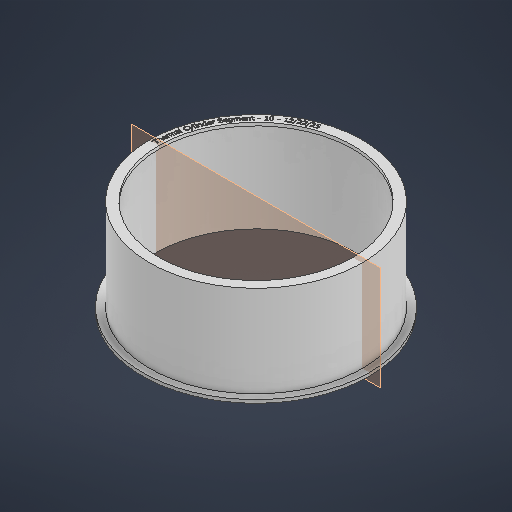
# Autodesk Inventor part: 10
Saved by Autodesk Inventor 2026.2 (Build 302298000, 298)
## iProperties
Created: 2024-04-11
Part Number: 10
Material: Generic
Document SubType Name: Modeling
Designer: Thienan Hoang
Density: 1 g/cm^3
Appearance: Default
Author: Thienan Hoang
Autodesk Inventor part; units mm, degrees
ref_plane "YZ Plane" through (0, 0, 0) normal (1, 0, 0) x (0, 1, 0)
ref_plane "XZ Plane" through (0, 0, 0) normal (0, 1, 0) x (-1, 0, 0)
sketch "Sketch1" plane through (0, 0, 0) normal (0, 1, 0) x (-1, 0, 0)
  circle A0 centre (0, 0) radius 72
  circle A1 centre (0, 0) radius 67.5
  circle A2 centre (0, 0) radius 63.5
  dimension "Absolute_Diameter" = 144
  dimension "Diameter_No_Outer_Lip" = 135
  dimension "Inner_Cylinder_Diameter" = 127
  constraints: 3 centre point, 3 coincident
  measures "Absolute_Diameter" diameter of A0
  measures "Diameter_No_Outer_Lip" diameter of A1
  measures "Inner_Cylinder_Diameter" diameter of A2
extrude "Extrusion1" add sketch "Sketch1" along normal blind 2 contours A0
extrude "Extrusion2" add sketch "Sketch1" along normal blind 60 contours A1
sketch "Sketch2" plane through (0, 60, 0) normal (0, 1, 0) x (1, 0, 0)
  circle A0 centre (0, 0) radius 61.5
  circle A1 centre (0, 0) radius 66.5
  dimension "Lip_Diameter_Out" = 123
  dimension "Top_Outer_Lip_Diameter" = 133
  constraints: 2 centre point, 2 coincident
  measures "Lip_Diameter_Out" diameter of A0
  measures "Top_Outer_Lip_Diameter" diameter of A1
extrude "Extrusion7" add sketch "Sketch2" against normal blind 2
ref_plane "Work Plane2" through (0, 10, 0) normal (0, 1, 0) x (1, 0, 0)
sketch "Sketch3" plane through (0, 10, 0) normal (0, 1, 0) x (1, 0, 0)
  circle A0 centre (0, 0) radius 127.5
  circle A1 centre (-127.5, 0) radius 2.5
  circle A2 centre (-103.1497, -74.9426) radius 2.5
  circle A3 centre (-39.3997, -121.2597) radius 2.5
  circle A4 centre (39.3997, -121.2597) radius 2.5
  circle A5 centre (103.1497, -74.9426) radius 2.5
  circle A6 centre (127.5, 0) radius 2.5
  circle A7 centre (103.1497, 74.9426) radius 2.5
  circle A8 centre (39.3997, 121.2597) radius 2.5
  circle A9 centre (-39.3997, 121.2597) radius 2.5
  circle A10 centre (-103.1497, 74.9426) radius 2.5
  dimension "d27" = 255
  dimension "d28" = 5
  dimension "d31" = 360
  constraints: 10 centre point, 1 coincident, 1 horizontal alignment, 23 other
  measures "d28" diameter of A1
extrude "Extrusion8" [suppressed]
sketch "Sketch24" plane through (0, 60, 0) normal (0, 1, 0) x (1, 0, 0)
  circle A0 centre (0, 0) radius 51
  circle A1 centre (0, -51) radius 2.75
  circle A2 centre (44.1673, -25.5) radius 2.75
  circle A3 centre (44.1673, 25.5) radius 2.75
  circle A4 centre (0, 51) radius 2.75
  circle A5 centre (-44.1673, 25.5) radius 2.75
  circle A6 centre (-44.1673, -25.5) radius 2.75
  dimension "d230" = 102
  dimension "d231" = 5.5
  dimension "d234" = 360
  constraints: 6 centre point, 1 coincident, 1 vertical alignment, 15 other
  measures "d231" diameter of A1
extrude "Extrusion30" [suppressed]
sketch "Sketch48" plane through (0, 60, 0) normal (0, 1, 0) x (1, 0, 0)
  circle A0 centre (0, 0) radius 58.25
  line L0 (-63.2421, 1.0199) -> (-65.929, 1.072)
  line L1 (-65.929, 1.072) -> (-65.9488, 0.0496)
  line L2 (-65.9488, 0.0496) -> (-66.3093, 0.0566)
  line L3 (-66.3093, 0.0566) -> (-66.2619, 2.5064)
  line L4 (-66.2619, 2.5064) -> (-65.9013, 2.4994)
  line L5 (-65.9013, 2.4994) -> (-65.9211, 1.477)
  line L6 (-65.9211, 1.477) -> (-63.2343, 1.4249)
  line L7 (-63.2343, 1.4249) -> (-63.2421, 1.0199)
  line L8 (-63.0947, 4.5212) -> (-63.1167, 4.1365)
  line L9 (-63.1167, 4.1365) -> (-64.4188, 4.211)
  spline S0 degree 2 poles (-64.4188, 4.211) (-64.5766, 4.2201) (-64.8496, 4.206) (-64.9335, 4.1663) knots 0 0 0 1 2 2 2
  spline S1 degree 2 poles (-64.9335, 4.1663) (-65.0225, 4.1244) (-65.1159, 3.9615) (-65.1241, 3.8185) knots 0 0 0 1 2 2 2
  spline S2 degree 2 poles (-65.1241, 3.8185) (-65.1323, 3.6754) (-64.9968, 3.3634) (-64.8818, 3.2108) knots 0 0 0 1 2 2 2
  line L10 (-64.8818, 3.2108) -> (-63.1754, 3.1131)
  line L11 (-63.1754, 3.1131) -> (-63.1974, 2.7284)
  line L12 (-63.1974, 2.7284) -> (-66.376, 2.9104)
  line L13 (-66.376, 2.9104) -> (-66.354, 3.2951)
  line L14 (-66.354, 3.2951) -> (-65.2048, 3.2293)
  spline S3 degree 2 poles (-65.2048, 3.2293) (-65.3503, 3.4108) (-65.494, 3.7531) (-65.4833, 3.9405) knots 0 0 0 1 2 2 2
  spline S4 degree 2 poles (-65.4833, 3.9405) (-65.4641, 4.2759) (-64.9984, 4.6302) (-64.5768, 4.606) knots 0 0 0 1 2 2 2
  line L15 (-64.5768, 4.606) -> (-63.0947, 4.5212)
  spline S5 degree 2 poles (-62.9087, 6.0442) (-62.9596, 5.4982) (-63.628, 4.9553) (-64.1937, 5.0082) knots 0 0 0 1 2 2 2
  spline S6 degree 2 poles (-64.1937, 5.0082) (-64.7495, 5.0601) (-65.3542, 5.7045) (-65.3103, 6.1742) knots 0 0 0 1 2 2 2
  spline S7 degree 2 poles (-65.3103, 6.1742) (-65.2906, 6.3857) (-65.137, 6.7013) (-64.9955, 6.8096) knots 0 0 0 1 2 2 2
  spline S8 degree 2 poles (-64.9955, 6.8096) (-64.8536, 6.9204) (-64.4652, 7.0156) (-64.1922, 6.9902) knots 0 0 0 1 2 2 2
  line L16 (-64.1922, 6.9902) -> (-63.9832, 6.9706)
  line L17 (-63.9832, 6.9706) -> (-64.1304, 5.3942)
  spline S9 degree 2 poles (-64.1304, 5.3942) (-63.7344, 5.3572) (-63.2767, 5.7164) (-63.2436, 6.0705) knots 0 0 0 1 2 2 2
  spline S10 degree 2 poles (-63.2436, 6.0705) (-63.2319, 6.1959) (-63.2657, 6.4447) (-63.3008, 6.5472) knots 0 0 0 1 2 2 2
  spline S11 degree 2 poles (-63.3008, 6.5472) (-63.3403, 6.6551) (-63.4131, 6.8058) (-63.4481, 6.8562) knots 0 0 0 1 2 2 2
  line L18 (-63.4481, 6.8562) -> (-63.446, 6.8783)
  line L19 (-63.446, 6.8783) -> (-63.0279, 6.8393)
  spline S12 degree 2 poles (-63.0279, 6.8393) (-63.0071, 6.7703) (-62.9472, 6.5613) (-62.9324, 6.4806) knots 0 0 0 1 2 2 2
  spline S13 degree 2 poles (-62.9324, 6.4806) (-62.9108, 6.3669) (-62.8958, 6.1819) (-62.9087, 6.0442) knots 0 0 0 1 2 2 2
  spline S14 degree 2 poles (-64.3107, 6.6241) (-64.4661, 6.6337) (-64.6983, 6.5909) (-64.7803, 6.5365) knots 0 0 0 1 2 2 2
  spline S15 degree 2 poles (-64.7803, 6.5365) (-64.8726, 6.4782) (-64.9831, 6.2776) (-64.9976, 6.1227) knots 0 0 0 1 2 2 2
  spline S16 degree 2 poles (-64.9976, 6.1227) (-65.0118, 5.9702) (-64.9408, 5.7477) (-64.8605, 5.6509) knots 0 0 0 1 2 2 2
  spline S17 degree 2 poles (-64.8605, 5.6509) (-64.7776, 5.5564) (-64.567, 5.4474) (-64.423, 5.4215) knots 0 0 0 1 2 2 2
  line L20 (-64.423, 5.4215) -> (-64.3107, 6.6241)
  line L21 (-64.5468, 8.6879) -> (-64.5493, 8.6683)
  spline S18 degree 2 poles (-64.5493, 8.6683) (-64.5669, 8.6256) (-64.5836, 8.5306) (-64.5918, 8.4644) knots 0 0 0 1 2 2 2
  spline S19 degree 2 poles (-64.5918, 8.4644) (-64.6108, 8.31) (-64.5134, 7.9894) (-64.3979, 7.8358) knots 0 0 0 1 2 2 2
  line L22 (-64.3979, 7.8358) -> (-62.7873, 7.6375)
  line L23 (-62.7873, 7.6375) -> (-62.8343, 7.2551)
  line L24 (-62.8343, 7.2551) -> (-65.1044, 7.5346)
  line L25 (-65.1044, 7.5346) -> (-65.0573, 7.917)
  line L26 (-65.0573, 7.917) -> (-64.719, 7.8754)
  spline S20 degree 2 poles (-64.719, 7.8754) (-64.8797, 8.1067) (-64.9934, 8.4367) (-64.9753, 8.5838) knots 0 0 0 1 2 2 2
  spline S21 degree 2 poles (-64.9753, 8.5838) (-64.968, 8.6427) (-64.9559, 8.7009) (-64.944, 8.7368) knots 0 0 0 1 2 2 2
  line L27 (-64.944, 8.7368) -> (-64.5468, 8.6879)
  line L28 (-62.2395, 11.316) -> (-63.546, 11.5299)
  spline S22 degree 2 poles (-63.546, 11.5299) (-63.702, 11.5554) (-63.9717, 11.5745) (-64.0512, 11.5475) knots 0 0 0 1 2 2 2
  spline S23 degree 2 poles (-64.0512, 11.5475) (-64.138, 11.5217) (-64.2404, 11.3857) (-64.2615, 11.2565) knots 0 0 0 1 2 2 2
  spline S24 degree 2 poles (-64.2615, 11.2565) (-64.2807, 11.1395) (-64.1807, 10.8479) (-64.0674, 10.6841) knots 0 0 0 1 2 2 2
  spline S25 degree 2 poles (-64.0674, 10.6841) (-64.0328, 10.681) (-63.937, 10.6703) (-63.8736, 10.6599) knots 0 0 0 1 2 2 2
  line L29 (-63.8736, 10.6599) -> (-62.3867, 10.4165)
  line L30 (-62.3867, 10.4165) -> (-62.4489, 10.0363)
  line L31 (-62.4489, 10.0363) -> (-63.7555, 10.2501)
  spline S26 degree 2 poles (-63.7555, 10.2501) (-63.9115, 10.2757) (-64.1812, 10.2948) (-64.2607, 10.2678) knots 0 0 0 1 2 2 2
  spline S27 degree 2 poles (-64.2607, 10.2678) (-64.3475, 10.2419) (-64.4498, 10.106) (-64.471, 9.9768) knots 0 0 0 1 2 2 2
  spline S28 degree 2 poles (-64.471, 9.9768) (-64.4909, 9.8549) (-64.3817, 9.5592) (-64.283, 9.4129) knots 0 0 0 1 2 2 2
  line L32 (-64.283, 9.4129) -> (-62.5962, 9.1368)
  line L33 (-62.5962, 9.1368) -> (-62.6584, 8.7565)
  line L34 (-62.6584, 8.7565) -> (-64.9156, 9.126)
  line L35 (-64.9156, 9.126) -> (-64.8534, 9.5063)
  line L36 (-64.8534, 9.5063) -> (-64.6047, 9.4656)
  spline S29 degree 2 poles (-64.6047, 9.4656) (-64.7291, 9.6386) (-64.8445, 9.9579) (-64.8158, 10.1334) knots 0 0 0 1 2 2 2
  spline S30 degree 2 poles (-64.8158, 10.1334) (-64.7831, 10.3333) (-64.5496, 10.6129) (-64.3292, 10.6594) knots 0 0 0 1 2 2 2
  spline S31 degree 2 poles (-64.3292, 10.6594) (-64.4935, 10.864) (-64.6374, 11.223) (-64.6063, 11.4131) knots 0 0 0 1 2 2 2
  spline S32 degree 2 poles (-64.6063, 11.4131) (-64.5824, 11.5594) (-64.4531, 11.7835) (-64.3363, 11.8545) knots 0 0 0 1 2 2 2
  spline S33 degree 2 poles (-64.3363, 11.8545) (-64.2192, 11.9279) (-63.8957, 11.9776) (-63.6641, 11.9396) knots 0 0 0 1 2 2 2
  line L37 (-63.6641, 11.9396) -> (-62.1772, 11.6962)
  line L38 (-62.1772, 11.6962) -> (-62.2395, 11.316)
  spline S34 degree 2 poles (-62.0371, 13.522) (-62.0129, 13.4689) (-61.9246, 13.2888) (-61.9037, 13.2087) knots 0 0 0 1 2 2 2
  spline S35 degree 2 poles (-61.9037, 13.2087) (-61.8713, 13.0984) (-61.8549, 12.9006) (-61.8905, 12.7314) knots 0 0 0 1 2 2 2
  spline S36 degree 2 poles (-61.8905, 12.7314) (-61.9195, 12.5936) (-62.0759, 12.3665) (-62.19, 12.2921) knots 0 0 0 1 2 2 2
  spline S37 degree 2 poles (-62.19, 12.2921) (-62.3007, 12.222) (-62.5943, 12.1702) (-62.7441, 12.2018) knots 0 0 0 1 2 2 2
  spline S38 degree 2 poles (-62.7441, 12.2018) (-62.9762, 12.2506) (-63.2637, 12.5156) (-63.3132, 12.7481) knots 0 0 0 1 2 2 2
  spline S39 degree 2 poles (-63.3132, 12.7481) (-63.3605, 12.955) (-63.3179, 13.4811) (-63.2722, 13.782) knots 0 0 0 1 2 2 2
  line L39 (-63.2722, 13.782) -> (-63.3447, 13.7972)
  spline S40 degree 2 poles (-63.3447, 13.7972) (-63.4753, 13.8247) (-63.654, 13.7791) (-63.7152, 13.7162) knots 0 0 0 1 2 2 2
  spline S41 degree 2 poles (-63.7152, 13.7162) (-63.7764, 13.6534) (-63.8491, 13.4516) (-63.8725, 13.3404) knots 0 0 0 1 2 2 2
  spline S42 degree 2 poles (-63.8725, 13.3404) (-63.9, 13.2099) (-63.8969, 12.8407) (-63.8591, 12.6485) knots 0 0 0 1 2 2 2
  line L40 (-63.8591, 12.6485) -> (-63.8637, 12.6268)
  line L41 (-63.8637, 12.6268) -> (-64.248, 12.7077)
  spline S43 degree 2 poles (-64.248, 12.7077) (-64.2552, 12.8177) (-64.2458, 13.2221) (-64.2056, 13.413) knots 0 0 0 1 2 2 2
  spline S44 degree 2 poles (-64.2056, 13.413) (-64.1567, 13.6451) (-64.0176, 13.9465) (-63.8968, 14.0523) knots 0 0 0 1 2 2 2
  spline S45 degree 2 poles (-63.8968, 14.0523) (-63.779, 14.1562) (-63.4611, 14.2155) (-63.2509, 14.1713) knots 0 0 0 1 2 2 2
  line L42 (-63.2509, 14.1713) -> (-61.7209, 13.8492)
  line L43 (-61.7209, 13.8492) -> (-61.8002, 13.4721)
  line L44 (-61.8002, 13.4721) -> (-62.0371, 13.522)
  line L45 (-62.3513, 13.5881) -> (-62.9725, 13.7189)
  spline S46 degree 2 poles (-62.9725, 13.7189) (-62.9889, 13.581) (-63.0338, 13.1639) (-63.0221, 13.0276) knots 0 0 0 1 2 2 2
  spline S47 degree 2 poles (-63.0221, 13.0276) (-63.0077, 12.8681) (-62.858, 12.6321) (-62.6888, 12.5965) knots 0 0 0 1 2 2 2
  spline S48 degree 2 poles (-62.6888, 12.5965) (-62.4954, 12.5558) (-62.2539, 12.7321) (-62.2101, 12.94) knots 0 0 0 1 2 2 2
  spline S49 degree 2 poles (-62.2101, 12.94) (-62.173, 13.1164) (-62.2642, 13.4385) (-62.3513, 13.5881) knots 0 0 0 1 2 2 2
  line L46 (-61.5046, 14.7574) -> (-61.5934, 14.3825)
  line L47 (-61.5934, 14.3825) -> (-64.6916, 15.1159)
  line L48 (-64.6916, 15.1159) -> (-64.6028, 15.4909)
  line L49 (-64.6028, 15.4909) -> (-61.5046, 14.7574)
  spline S50 degree 2 poles (-60.6572, 17.7329) (-60.7393, 17.4481) (-61.0704, 17.0217) (-61.3132, 16.9015) knots 0 0 0 1 2 2 2
  spline S51 degree 2 poles (-61.3132, 16.9015) (-61.5537, 16.7806) (-62.1788, 16.7525) (-62.549, 16.8592) knots 0 0 0 1 2 2 2
  spline S52 degree 2 poles (-62.549, 16.8592) (-62.9169, 16.9652) (-63.4087, 17.3101) (-63.5592, 17.5462) knots 0 0 0 1 2 2 2
  spline S53 degree 2 poles (-63.5592, 17.5462) (-63.7055, 17.7786) (-63.7739, 18.3176) (-63.6883, 18.6142) knots 0 0 0 1 2 2 2
  spline S54 degree 2 poles (-63.6883, 18.6142) (-63.6459, 18.7614) (-63.5287, 19.0078) (-63.464, 19.1074) knots 0 0 0 1 2 2 2
  spline S55 degree 2 poles (-63.464, 19.1074) (-63.4057, 19.1934) (-63.2611, 19.3651) (-63.1809, 19.4474) knots 0 0 0 1 2 2 2
  line L50 (-63.1809, 19.4474) -> (-62.711, 19.3119)
  line L51 (-62.711, 19.3119) -> (-62.7198, 19.2811)
  spline S56 degree 2 poles (-62.7198, 19.2811) (-62.7824, 19.2425) (-62.9618, 19.1194) (-63.0594, 19.0216) knots 0 0 0 1 2 2 2
  spline S57 degree 2 poles (-63.0594, 19.0216) (-63.1532, 18.9278) (-63.3075, 18.687) (-63.3568, 18.5161) knots 0 0 0 1 2 2 2
  spline S58 degree 2 poles (-63.3568, 18.5161) (-63.4108, 18.3286) (-63.353, 17.9495) (-63.2421, 17.7813) knots 0 0 0 1 2 2 2
  spline S59 degree 2 poles (-63.2421, 17.7813) (-63.1281, 17.6148) (-62.7145, 17.3464) (-62.432, 17.265) knots 0 0 0 1 2 2 2
  spline S60 degree 2 poles (-62.432, 17.265) (-62.1306, 17.1782) (-61.6546, 17.1978) (-61.4688, 17.2805) knots 0 0 0 1 2 2 2
  spline S61 degree 2 poles (-61.4688, 17.2805) (-61.2884, 17.3622) (-61.0462, 17.6496) (-60.9928, 17.8348) knots 0 0 0 1 2 2 2
  spline S62 degree 2 poles (-60.9928, 17.8348) (-60.9443, 18.0033) (-60.9446, 18.3144) (-60.9741, 18.4437) knots 0 0 0 1 2 2 2
  spline S63 degree 2 poles (-60.9741, 18.4437) (-61.0051, 18.5683) (-61.0874, 18.7643) (-61.1195, 18.8224) knots 0 0 0 1 2 2 2
  line L52 (-61.1195, 18.8224) -> (-61.1113, 18.8509)
  line L53 (-61.1113, 18.8509) -> (-60.6461, 18.7168)
  spline S64 degree 2 poles (-60.6461, 18.7168) (-60.629, 18.6065) (-60.5952, 18.4117) (-60.5921, 18.2797) knots 0 0 0 1 2 2 2
  spline S65 degree 2 poles (-60.5921, 18.2797) (-60.5864, 18.1392) (-60.6066, 17.9085) (-60.6572, 17.7329) knots 0 0 0 1 2 2 2
  line L54 (-61.9503, 21.409) -> (-59.3602, 19.2647)
  line L55 (-59.3602, 19.2647) -> (-59.4888, 18.8728)
  line L56 (-59.4888, 18.8728) -> (-60.2669, 19.5596)
  line L57 (-60.2669, 19.5596) -> (-62.5933, 19.4493)
  line L58 (-62.5933, 19.4493) -> (-62.4639, 19.8436)
  line L59 (-62.4639, 19.8436) -> (-60.6591, 19.9092)
  line L60 (-60.6591, 19.9092) -> (-62.0751, 21.0288)
  line L61 (-62.0751, 21.0288) -> (-61.9503, 21.409)
  line L62 (-59.5421, 21.3387) -> (-59.671, 20.9756)
  line L63 (-59.671, 20.9756) -> (-62.6714, 22.0406)
  line L64 (-62.6714, 22.0406) -> (-62.5425, 22.4037)
  line L65 (-62.5425, 22.4037) -> (-59.5421, 21.3387)
  line L66 (-59.2119, 22.2384) -> (-59.3463, 21.8773)
  line L67 (-59.3463, 21.8773) -> (-61.49, 22.6749)
  line L68 (-61.49, 22.6749) -> (-61.3556, 23.036)
  line L69 (-61.3556, 23.036) -> (-59.2119, 22.2384)
  line L70 (-61.7026, 23.1942) -> (-61.8551, 22.7844)
  line L71 (-61.8551, 22.7844) -> (-62.2301, 22.924)
  line L72 (-62.2301, 22.924) -> (-62.0776, 23.3337)
  line L73 (-62.0776, 23.3337) -> (-61.7026, 23.1942)
  line L74 (-58.3464, 24.4352) -> (-58.4902, 24.0777)
  line L75 (-58.4902, 24.0777) -> (-59.7002, 24.5642)
  spline S66 degree 2 poles (-59.7002, 24.5642) (-59.8469, 24.6231) (-60.11, 24.697) (-60.2022, 24.6861) knots 0 0 0 1 2 2 2
  spline S67 degree 2 poles (-60.2022, 24.6861) (-60.3, 24.6748) (-60.4405, 24.5503) (-60.494, 24.4174) knots 0 0 0 1 2 2 2
  spline S68 degree 2 poles (-60.494, 24.4174) (-60.5474, 24.2845) (-60.5186, 23.9455) (-60.4584, 23.7642) knots 0 0 0 1 2 2 2
  line L76 (-60.4584, 23.7642) -> (-58.8725, 23.1266)
  line L77 (-58.8725, 23.1266) -> (-59.0163, 22.7691)
  line L78 (-59.0163, 22.7691) -> (-61.1384, 23.6223)
  line L79 (-61.1384, 23.6223) -> (-60.9947, 23.9798)
  line L80 (-60.9947, 23.9798) -> (-60.7586, 23.8849)
  spline S69 degree 2 poles (-60.7586, 23.8849) (-60.8385, 24.1034) (-60.8654, 24.4736) (-60.7954, 24.6477) knots 0 0 0 1 2 2 2
  spline S70 degree 2 poles (-60.7954, 24.6477) (-60.6701, 24.9594) (-60.1156, 25.1465) (-59.7238, 24.9889) knots 0 0 0 1 2 2 2
  line L81 (-59.7238, 24.9889) -> (-58.3464, 24.4352)
  line L82 (-57.4194, 26.5395) -> (-57.5762, 26.1875)
  line L83 (-57.5762, 26.1875) -> (-57.7883, 26.282)
  spline S71 degree 2 poles (-57.7883, 26.282) (-57.7568, 26.1706) (-57.7198, 26.0108) (-57.7177, 25.9125) knots 0 0 0 1 2 2 2
  spline S72 degree 2 poles (-57.7177, 25.9125) (-57.7147, 25.822) (-57.7477, 25.6447) (-57.795, 25.5386) knots 0 0 0 1 2 2 2
  spline S73 degree 2 poles (-57.795, 25.5386) (-57.8713, 25.3671) (-58.1421, 25.1417) (-58.325, 25.1014) knots 0 0 0 1 2 2 2
  spline S74 degree 2 poles (-58.325, 25.1014) (-58.5079, 25.0612) (-58.9642, 25.1293) (-59.2282, 25.2469) knots 0 0 0 1 2 2 2
  spline S75 degree 2 poles (-59.2282, 25.2469) (-59.5035, 25.3695) (-59.8418, 25.6905) (-59.9377, 25.882) knots 0 0 0 1 2 2 2
  spline S76 degree 2 poles (-59.9377, 25.882) (-60.0218, 26.0574) (-60.0338, 26.4494) (-59.9544, 26.6276) knots 0 0 0 1 2 2 2
  spline S77 degree 2 poles (-59.9544, 26.6276) (-59.885, 26.7833) (-59.7116, 26.9845) (-59.5821, 27.081) knots 0 0 0 1 2 2 2
  line L84 (-59.5821, 27.081) -> (-60.4846, 27.483)
  line L85 (-60.4846, 27.483) -> (-60.3278, 27.835)
  line L86 (-60.3278, 27.835) -> (-57.4194, 26.5395)
  line L87 (-58.0839, 26.4136) -> (-59.291, 26.9513)
  spline S78 degree 2 poles (-59.291, 26.9513) (-59.4125, 26.8486) (-59.5523, 26.6621) (-59.6056, 26.5425) knots 0 0 0 1 2 2 2
  spline S79 degree 2 poles (-59.6056, 26.5425) (-59.7262, 26.2718) (-59.4568, 25.784) (-59.0732, 25.6132) knots 0 0 0 1 2 2 2
  spline S80 degree 2 poles (-59.0732, 25.6132) (-58.7031, 25.4483) (-58.2083, 25.5091) (-58.0927, 25.7686) knots 0 0 0 1 2 2 2
  spline S81 degree 2 poles (-58.0927, 25.7686) (-58.0314, 25.9062) (-58.0331, 26.2423) (-58.0839, 26.4136) knots 0 0 0 1 2 2 2
  spline S82 degree 2 poles (-56.6996, 27.914) (-56.9405, 27.4214) (-57.7577, 27.1501) (-58.2681, 27.3997) knots 0 0 0 1 2 2 2
  spline S83 degree 2 poles (-58.2681, 27.3997) (-58.7696, 27.6449) (-59.1071, 28.4616) (-58.8998, 28.8854) knots 0 0 0 1 2 2 2
  spline S84 degree 2 poles (-58.8998, 28.8854) (-58.8065, 29.0762) (-58.5513, 29.3171) (-58.3805, 29.3683) knots 0 0 0 1 2 2 2
  spline S85 degree 2 poles (-58.3805, 29.3683) (-58.2086, 29.4218) (-57.8116, 29.3734) (-57.5653, 29.2529) knots 0 0 0 1 2 2 2
  line L88 (-57.5653, 29.2529) -> (-57.3767, 29.1607)
  line L89 (-57.3767, 29.1607) -> (-58.0722, 27.7383)
  spline S86 degree 2 poles (-58.0722, 27.7383) (-57.715, 27.5637) (-57.1598, 27.7376) (-57.0035, 28.0571) knots 0 0 0 1 2 2 2
  spline S87 degree 2 poles (-57.0035, 28.0571) (-56.9482, 28.1703) (-56.8918, 28.4149) (-56.8883, 28.5232) knots 0 0 0 1 2 2 2
  spline S88 degree 2 poles (-56.8883, 28.5232) (-56.8871, 28.6381) (-56.9019, 28.8048) (-56.9168, 28.8643) knots 0 0 0 1 2 2 2
  line L90 (-56.9168, 28.8643) -> (-56.907, 28.8843)
  line L91 (-56.907, 28.8843) -> (-56.5298, 28.6998)
  spline S89 degree 2 poles (-56.5298, 28.6998) (-56.5347, 28.6279) (-56.5526, 28.4113) (-56.5674, 28.3305) knots 0 0 0 1 2 2 2
  spline S90 degree 2 poles (-56.5674, 28.3305) (-56.5874, 28.2165) (-56.6388, 28.0382) (-56.6996, 27.914) knots 0 0 0 1 2 2 2
  spline S91 degree 2 poles (-57.8057, 28.9525) (-57.9477, 29.0164) (-58.18, 29.0586) (-58.2759, 29.0367) knots 0 0 0 1 2 2 2
  spline S92 degree 2 poles (-58.2759, 29.0367) (-58.3829, 29.0148) (-58.5572, 28.8663) (-58.6256, 28.7265) knots 0 0 0 1 2 2 2
  spline S93 degree 2 poles (-58.6256, 28.7265) (-58.6928, 28.589) (-58.7051, 28.3558) (-58.6643, 28.2368) knots 0 0 0 1 2 2 2
  spline S94 degree 2 poles (-58.6643, 28.2368) (-58.6202, 28.119) (-58.4618, 27.9426) (-58.3363, 27.8675) knots 0 0 0 1 2 2 2
  line L92 (-58.3363, 27.8675) -> (-57.8057, 28.9525)
  line L93 (-57.2963, 30.9663) -> (-57.3055, 30.9488)
  spline S95 degree 2 poles (-57.3055, 30.9488) (-57.3371, 30.9152) (-57.3863, 30.8322) (-57.4174, 30.7732) knots 0 0 0 1 2 2 2
  spline S96 degree 2 poles (-57.4174, 30.7732) (-57.4898, 30.6355) (-57.5121, 30.3012) (-57.4585, 30.1167) knots 0 0 0 1 2 2 2
  line L94 (-57.4585, 30.1167) -> (-56.0222, 29.3613)
  line L95 (-56.0222, 29.3613) -> (-56.2016, 29.0202)
  line L96 (-56.2016, 29.0202) -> (-58.2259, 30.0849)
  line L97 (-58.2259, 30.0849) -> (-58.0465, 30.4259)
  line L98 (-58.0465, 30.4259) -> (-57.7448, 30.2673)
  spline S97 degree 2 poles (-57.7448, 30.2673) (-57.8133, 30.5405) (-57.8028, 30.8894) (-57.7338, 31.0206) knots 0 0 0 1 2 2 2
  spline S98 degree 2 poles (-57.7338, 31.0206) (-57.7062, 31.073) (-57.6742, 31.1232) (-57.6504, 31.1525) knots 0 0 0 1 2 2 2
  line L99 (-57.6504, 31.1525) -> (-57.2963, 30.9663)
  spline S99 degree 2 poles (-54.3606, 32.2276) (-54.5294, 31.943) (-54.8852, 31.6141) (-55.0748, 31.4882) knots 0 0 0 1 2 2 2
  line L100 (-55.0748, 31.4882) -> (-55.5124, 31.7477)
  line L101 (-55.5124, 31.7477) -> (-55.4973, 31.7732)
  spline S100 degree 2 poles (-55.4973, 31.7732) (-55.2338, 31.8495) (-54.7971, 32.1792) (-54.6774, 32.3811) knots 0 0 0 1 2 2 2
  spline S101 degree 2 poles (-54.6774, 32.3811) (-54.506, 32.67) (-54.571, 33.1077) (-54.7685, 33.2248) knots 0 0 0 1 2 2 2
  spline S102 degree 2 poles (-54.7685, 33.2248) (-54.9258, 33.3181) (-55.2132, 33.2789) (-55.3616, 33.14) knots 0 0 0 1 2 2 2
  spline S103 degree 2 poles (-55.3616, 33.14) (-55.4674, 33.0391) (-55.6338, 32.865) (-55.7615, 32.7368) knots 0 0 0 1 2 2 2
  spline S104 degree 2 poles (-55.7615, 32.7368) (-55.8783, 32.6223) (-56.1139, 32.472) (-56.2501, 32.4408) knots 0 0 0 1 2 2 2
  spline S105 degree 2 poles (-56.2501, 32.4408) (-56.3851, 32.4117) (-56.6717, 32.461) (-56.8247, 32.5518) knots 0 0 0 1 2 2 2
  spline S106 degree 2 poles (-56.8247, 32.5518) (-57.1433, 32.7407) (-57.2798, 33.4936) (-57.0518, 33.8782) knots 0 0 0 1 2 2 2
  spline S107 degree 2 poles (-57.0518, 33.8782) (-56.9207, 34.0991) (-56.6018, 34.4384) (-56.4194, 34.5571) knots 0 0 0 1 2 2 2
  line L102 (-56.4194, 34.5571) -> (-56.003, 34.3101)
  line L103 (-56.003, 34.3101) -> (-56.0181, 34.2846)
  spline S108 degree 2 poles (-56.0181, 34.2846) (-56.2072, 34.2273) (-56.609, 33.9372) (-56.7362, 33.7226) knots 0 0 0 1 2 2 2
  spline S109 degree 2 poles (-56.7362, 33.7226) (-56.8798, 33.4804) (-56.8302, 33.0461) (-56.6453, 32.9365) knots 0 0 0 1 2 2 2
  spline S110 degree 2 poles (-56.6453, 32.9365) (-56.4796, 32.8382) (-56.1775, 32.8974) (-56.0346, 33.0366) knots 0 0 0 1 2 2 2
  spline S111 degree 2 poles (-56.0346, 33.0366) (-55.9393, 33.1294) (-55.6726, 33.4049) (-55.5777, 33.4922) knots 0 0 0 1 2 2 2
  spline S112 degree 2 poles (-55.5777, 33.4922) (-55.3349, 33.7129) (-54.8526, 33.7658) (-54.6083, 33.6209) knots 0 0 0 1 2 2 2
  spline S113 degree 2 poles (-54.6083, 33.6209) (-54.4532, 33.5289) (-54.2301, 33.2272) (-54.1928, 33.0529) knots 0 0 0 1 2 2 2
  spline S114 degree 2 poles (-54.1928, 33.0529) (-54.1524, 32.8595) (-54.2182, 32.4677) (-54.3606, 32.2276) knots 0 0 0 1 2 2 2
  spline S115 degree 2 poles (-53.0753, 34.3081) (-53.3717, 33.8468) (-54.2149, 33.6723) (-54.6929, 33.9794) knots 0 0 0 1 2 2 2
  spline S116 degree 2 poles (-54.6929, 33.9794) (-55.1625, 34.2812) (-55.4029, 35.1316) (-55.1479, 35.5284) knots 0 0 0 1 2 2 2
  spline S117 degree 2 poles (-55.1479, 35.5284) (-55.033, 35.7071) (-54.7515, 35.9167) (-54.576, 35.9478) knots 0 0 0 1 2 2 2
  spline S118 degree 2 poles (-54.576, 35.9478) (-54.3991, 35.9809) (-54.0104, 35.8867) (-53.7797, 35.7385) knots 0 0 0 1 2 2 2
  line L104 (-53.7797, 35.7385) -> (-53.6031, 35.625)
  line L105 (-53.6031, 35.625) -> (-54.459, 34.2931)
  spline S119 degree 2 poles (-54.459, 34.2931) (-54.1245, 34.0781) (-53.5528, 34.1864) (-53.3605, 34.4856) knots 0 0 0 1 2 2 2
  spline S120 degree 2 poles (-53.3605, 34.4856) (-53.2924, 34.5916) (-53.208, 34.828) (-53.192, 34.9351) knots 0 0 0 1 2 2 2
  spline S121 degree 2 poles (-53.192, 34.9351) (-53.1775, 35.0491) (-53.1728, 35.2164) (-53.1807, 35.2772) knots 0 0 0 1 2 2 2
  line L106 (-53.1807, 35.2772) -> (-53.1686, 35.2959)
  line L107 (-53.1686, 35.2959) -> (-52.8154, 35.0689)
  spline S122 degree 2 poles (-52.8154, 35.0689) (-52.8286, 34.9981) (-52.8716, 34.785) (-52.8956, 34.7065) knots 0 0 0 1 2 2 2
  spline S123 degree 2 poles (-52.8956, 34.7065) (-52.9287, 34.5956) (-53.0005, 34.4245) (-53.0753, 34.3081) knots 0 0 0 1 2 2 2
  spline S124 degree 2 poles (-54.0533, 35.4681) (-54.1869, 35.548) (-54.4128, 35.6169) (-54.5106, 35.6063) knots 0 0 0 1 2 2 2
  spline S125 degree 2 poles (-54.5106, 35.6063) (-54.6194, 35.5969) (-54.8098, 35.4697) (-54.8939, 35.3388) knots 0 0 0 1 2 2 2
  spline S126 degree 2 poles (-54.8939, 35.3388) (-54.9767, 35.21) (-55.016, 34.9798) (-54.9892, 34.8569) knots 0 0 0 1 2 2 2
  spline S127 degree 2 poles (-54.9892, 34.8569) (-54.9591, 34.7348) (-54.8222, 34.5411) (-54.7063, 34.452) knots 0 0 0 1 2 2 2
  line L108 (-54.7063, 34.452) -> (-54.0533, 35.4681)
  spline S128 degree 2 poles (-52.109, 35.2099) (-52.0723, 35.2325) (-51.9417, 35.3253) (-51.8685, 35.3917) knots 0 0 0 1 2 2 2
  spline S129 degree 2 poles (-51.8685, 35.3917) (-51.7856, 35.4635) (-51.6564, 35.5933) (-51.5958, 35.6805) knots 0 0 0 1 2 2 2
  spline S130 degree 2 poles (-51.5958, 35.6805) (-51.4944, 35.8266) (-51.4306, 36.083) (-51.4602, 36.1877) knots 0 0 0 1 2 2 2
  spline S131 degree 2 poles (-51.4602, 36.1877) (-51.4911, 36.2904) (-51.6421, 36.4584) (-51.7577, 36.5387) knots 0 0 0 1 2 2 2
  line L109 (-51.7577, 36.5387) -> (-51.9221, 36.6528)
  spline S132 degree 2 poles (-51.9221, 36.6528) (-51.8992, 36.4475) (-51.9642, 36.1287) (-52.0924, 35.9441) knots 0 0 0 1 2 2 2
  spline S133 degree 2 poles (-52.0924, 35.9441) (-52.315, 35.6236) (-53.0552, 35.5752) (-53.5036, 35.8865) knots 0 0 0 1 2 2 2
  spline S134 degree 2 poles (-53.5036, 35.8865) (-53.7369, 36.0485) (-54.0065, 36.4312) (-54.0582, 36.6295) knots 0 0 0 1 2 2 2
  spline S135 degree 2 poles (-54.0582, 36.6295) (-54.1047, 36.8181) (-54.0351, 37.1998) (-53.9281, 37.354) knots 0 0 0 1 2 2 2
  spline S136 degree 2 poles (-53.9281, 37.354) (-53.8266, 37.5001) (-53.6097, 37.6652) (-53.4722, 37.7291) knots 0 0 0 1 2 2 2
  line L110 (-53.4722, 37.7291) -> (-53.5386, 37.8023)
  line L111 (-53.5386, 37.8023) -> (-53.3315, 38.1005)
  line L112 (-53.3315, 38.1005) -> (-51.6678, 36.9454)
  spline S137 degree 2 poles (-51.6678, 36.9454) (-51.189, 36.6129) (-51.0314, 35.8871) (-51.3287, 35.459) knots 0 0 0 1 2 2 2
  spline S138 degree 2 poles (-51.3287, 35.459) (-51.4245, 35.321) (-51.6692, 35.0639) (-51.7916, 34.9655) knots 0 0 0 1 2 2 2
  line L113 (-51.7916, 34.9655) -> (-52.1203, 35.1937)
  line L114 (-52.1203, 35.1937) -> (-52.109, 35.2099)
  line L115 (-52.1818, 36.8331) -> (-53.2145, 37.5502)
  spline S139 degree 2 poles (-53.2145, 37.5502) (-53.353, 37.4719) (-53.5398, 37.3069) (-53.6088, 37.2075) knots 0 0 0 1 2 2 2
  spline S140 degree 2 poles (-53.6088, 37.2075) (-53.775, 36.9681) (-53.6136, 36.447) (-53.2829, 36.2174) knots 0 0 0 1 2 2 2
  spline S141 degree 2 poles (-53.2829, 36.2174) (-52.9704, 36.0005) (-52.4987, 35.9826) (-52.3353, 36.218) knots 0 0 0 1 2 2 2
  spline S142 degree 2 poles (-52.3353, 36.218) (-52.2493, 36.3418) (-52.1664, 36.6691) (-52.1818, 36.8331) knots 0 0 0 1 2 2 2
  line L116 (-49.5594, 39.315) -> (-50.6109, 40.1194)
  spline S143 degree 2 poles (-50.6109, 40.1194) (-50.7365, 40.2154) (-50.9653, 40.3594) (-51.0482, 40.3731) knots 0 0 0 1 2 2 2
  spline S144 degree 2 poles (-51.0482, 40.3731) (-51.1369, 40.3912) (-51.2913, 40.3195) (-51.3708, 40.2156) knots 0 0 0 1 2 2 2
  spline S145 degree 2 poles (-51.3708, 40.2156) (-51.4428, 40.1214) (-51.4922, 39.8171) (-51.4694, 39.6192) knots 0 0 0 1 2 2 2
  spline S146 degree 2 poles (-51.4694, 39.6192) (-51.4404, 39.6002) (-51.3609, 39.5456) (-51.3099, 39.5066) knots 0 0 0 1 2 2 2
  line L117 (-51.3099, 39.5066) -> (-50.1132, 38.5911)
  line L118 (-50.1132, 38.5911) -> (-50.3473, 38.285)
  line L119 (-50.3473, 38.285) -> (-51.3988, 39.0895)
  spline S147 degree 2 poles (-51.3988, 39.0895) (-51.5244, 39.1855) (-51.7532, 39.3295) (-51.8361, 39.3431) knots 0 0 0 1 2 2 2
  spline S148 degree 2 poles (-51.8361, 39.3431) (-51.9248, 39.3613) (-52.0792, 39.2896) (-52.1587, 39.1856) knots 0 0 0 1 2 2 2
  spline S149 degree 2 poles (-52.1587, 39.1856) (-52.2338, 39.0876) (-52.2768, 38.7752) (-52.2587, 38.5997) knots 0 0 0 1 2 2 2
  line L120 (-52.2587, 38.5997) -> (-50.9011, 37.5611)
  line L121 (-50.9011, 37.5611) -> (-51.1352, 37.2551)
  line L122 (-51.1352, 37.2551) -> (-52.9518, 38.6448)
  line L123 (-52.9518, 38.6448) -> (-52.7177, 38.9509)
  line L124 (-52.7177, 38.9509) -> (-52.5176, 38.7978)
  spline S150 degree 2 poles (-52.5176, 38.7978) (-52.5457, 39.009) (-52.4971, 39.345) (-52.389, 39.4862) knots 0 0 0 1 2 2 2
  spline S151 degree 2 poles (-52.389, 39.4862) (-52.266, 39.6471) (-51.9282, 39.7837) (-51.7119, 39.7209) knots 0 0 0 1 2 2 2
  spline S152 degree 2 poles (-51.7119, 39.7209) (-51.7604, 39.9787) (-51.7182, 40.3631) (-51.6011, 40.5162) knots 0 0 0 1 2 2 2
  spline S153 degree 2 poles (-51.6011, 40.5162) (-51.5111, 40.6339) (-51.2914, 40.7706) (-51.155, 40.7782) knots 0 0 0 1 2 2 2
  spline S154 degree 2 poles (-51.155, 40.7782) (-51.017, 40.7877) (-50.7083, 40.6791) (-50.522, 40.5365) knots 0 0 0 1 2 2 2
  line L125 (-50.522, 40.5365) -> (-49.3253, 39.621)
  line L126 (-49.3253, 39.621) -> (-49.5594, 39.315)
  spline S155 degree 2 poles (-48.2971, 40.7606) (-48.6496, 40.3406) (-49.5082, 40.2744) (-49.9433, 40.6396) knots 0 0 0 1 2 2 2
  spline S156 degree 2 poles (-49.9433, 40.6396) (-50.3709, 40.9985) (-50.5015, 41.8725) (-50.1982, 42.2338) knots 0 0 0 1 2 2 2
  spline S157 degree 2 poles (-50.1982, 42.2338) (-50.0617, 42.3965) (-49.7559, 42.5687) (-49.5778, 42.5773) knots 0 0 0 1 2 2 2
  spline S158 degree 2 poles (-49.5778, 42.5773) (-49.3981, 42.5877) (-49.0245, 42.445) (-48.8145, 42.2687) knots 0 0 0 1 2 2 2
  line L127 (-48.8145, 42.2687) -> (-48.6537, 42.1338)
  line L128 (-48.6537, 42.1338) -> (-49.6716, 40.9211)
  spline S159 degree 2 poles (-49.6716, 40.9211) (-49.367, 40.6654) (-48.7862, 40.7003) (-48.5576, 40.9728) knots 0 0 0 1 2 2 2
  spline S160 degree 2 poles (-48.5576, 40.9728) (-48.4766, 41.0692) (-48.3629, 41.2931) (-48.3334, 41.3973) knots 0 0 0 1 2 2 2
  spline S161 degree 2 poles (-48.3334, 41.3973) (-48.3045, 41.5085) (-48.2787, 41.6738) (-48.2788, 41.7352) knots 0 0 0 1 2 2 2
  line L129 (-48.2788, 41.7352) -> (-48.2645, 41.7522)
  line L130 (-48.2645, 41.7522) -> (-47.9428, 41.4823)
  spline S162 degree 2 poles (-47.9428, 41.4823) (-47.9649, 41.4137) (-48.0346, 41.2078) (-48.0684, 41.1329) knots 0 0 0 1 2 2 2
  spline S163 degree 2 poles (-48.0684, 41.1329) (-48.1152, 41.0272) (-48.2082, 40.8665) (-48.2971, 40.7606) knots 0 0 0 1 2 2 2
  spline S164 degree 2 poles (-49.1202, 42.0352) (-49.2426, 42.1314) (-49.4579, 42.2283) (-49.5562, 42.2303) knots 0 0 0 1 2 2 2
  spline S165 degree 2 poles (-49.5562, 42.2303) (-49.6653, 42.2348) (-49.8703, 42.1327) (-49.9704, 42.0135) knots 0 0 0 1 2 2 2
  spline S166 degree 2 poles (-49.9704, 42.0135) (-50.0688, 41.8962) (-50.137, 41.6729) (-50.126, 41.5476) knots 0 0 0 1 2 2 2
  spline S167 degree 2 poles (-50.126, 41.5476) (-50.1116, 41.4226) (-50.0004, 41.2132) (-49.8967, 41.11) knots 0 0 0 1 2 2 2
  line L131 (-49.8967, 41.11) -> (-49.1202, 42.0352)
  line L132 (-46.3473, 43.0501) -> (-46.6055, 42.764)
  line L133 (-46.6055, 42.764) -> (-47.5737, 43.6378)
  spline S168 degree 2 poles (-47.5737, 43.6378) (-47.691, 43.7437) (-47.9126, 43.9038) (-48.0029, 43.9254) knots 0 0 0 1 2 2 2
  spline S169 degree 2 poles (-48.0029, 43.9254) (-48.0985, 43.9485) (-48.2734, 43.88) (-48.3694, 43.7737) knots 0 0 0 1 2 2 2
  spline S170 degree 2 poles (-48.3694, 43.7737) (-48.4653, 43.6673) (-48.5552, 43.3392) (-48.5612, 43.1483) knots 0 0 0 1 2 2 2
  line L134 (-48.5612, 43.1483) -> (-47.2923, 42.0031)
  line L135 (-47.2923, 42.0031) -> (-47.5504, 41.717)
  line L136 (-47.5504, 41.717) -> (-49.2484, 43.2495)
  line L137 (-49.2484, 43.2495) -> (-48.9902, 43.5355)
  line L138 (-48.9902, 43.5355) -> (-48.8014, 43.365)
  spline S171 degree 2 poles (-48.8014, 43.365) (-48.801, 43.5977) (-48.6987, 43.9544) (-48.5729, 44.0938) knots 0 0 0 1 2 2 2
  spline S172 degree 2 poles (-48.5729, 44.0938) (-48.3478, 44.3432) (-47.7629, 44.3277) (-47.4493, 44.0447) knots 0 0 0 1 2 2 2
  line L139 (-47.4493, 44.0447) -> (-46.3473, 43.0501)
  spline S173 degree 2 poles (-45.4634, 43.9101) (-45.6803, 43.6835) (-46.1833, 43.6761) (-46.4634, 43.9443) knots 0 0 0 1 2 2 2
  line L140 (-46.4634, 43.9443) -> (-47.3785, 44.8207)
  line L141 (-47.3785, 44.8207) -> (-47.5579, 44.6334)
  line L142 (-47.5579, 44.6334) -> (-47.788, 44.8538)
  line L143 (-47.788, 44.8538) -> (-47.6087, 45.0411)
  line L144 (-47.6087, 45.0411) -> (-48.0832, 45.4955)
  line L145 (-48.0832, 45.4955) -> (-47.8167, 45.7738)
  line L146 (-47.8167, 45.7738) -> (-47.3422, 45.3194)
  line L147 (-47.3422, 45.3194) -> (-46.8519, 45.8314)
  line L148 (-46.8519, 45.8314) -> (-46.6217, 45.611)
  line L149 (-46.6217, 45.611) -> (-47.112, 45.099)
  line L150 (-47.112, 45.099) -> (-46.3253, 44.3456)
  spline S174 degree 2 poles (-46.3253, 44.3456) (-46.2004, 44.2261) (-46.0545, 44.1034) (-45.9666, 44.0774) knots 0 0 0 1 2 2 2
  spline S175 degree 2 poles (-45.9666, 44.0774) (-45.891, 44.0528) (-45.7316, 44.1157) (-45.6394, 44.212) knots 0 0 0 1 2 2 2
  spline S176 degree 2 poles (-45.6394, 44.212) (-45.5744, 44.2798) (-45.4942, 44.4457) (-45.4793, 44.4862) knots 0 0 0 1 2 2 2
  line L151 (-45.4793, 44.4862) -> (-45.464, 44.5023)
  line L152 (-45.464, 44.5023) -> (-45.2142, 44.2631)
  spline S177 degree 2 poles (-45.2142, 44.2631) (-45.268, 44.1641) (-45.3967, 43.9797) (-45.4634, 43.9101) knots 0 0 0 1 2 2 2
  line L153 (-44.098, 46.9348) -> (-44.9316, 46.1374)
  line L154 (-44.9316, 46.1374) -> (-45.1877, 46.4051)
  line L155 (-45.1877, 46.4051) -> (-44.3541, 47.2025)
  line L156 (-44.3541, 47.2025) -> (-44.098, 46.9348)
  line L157 (-40.735, 48.3929) -> (-41.8603, 47.4209)
  line L158 (-41.8603, 47.4209) -> (-42.0637, 47.6564)
  line L159 (-42.0637, 47.6564) -> (-41.645, 48.0181)
  line L160 (-41.645, 48.0181) -> (-42.9803, 49.564)
  line L161 (-42.9803, 49.564) -> (-43.399, 49.2023)
  line L162 (-43.399, 49.2023) -> (-43.5814, 49.4135)
  spline S178 degree 2 poles (-43.5814, 49.4135) (-43.344, 49.6186) (-43.236, 49.9469) (-43.3825, 50.1468) knots 0 0 0 1 2 2 2
  line L163 (-43.3825, 50.1468) -> (-43.1432, 50.3534)
  line L164 (-43.1432, 50.3534) -> (-41.3478, 48.2748)
  line L165 (-41.3478, 48.2748) -> (-40.9384, 48.6284)
  line L166 (-40.9384, 48.6284) -> (-40.735, 48.3929)
  spline S179 degree 2 poles (-39.7799, 51.1291) (-39.2666, 50.4895) (-39.1577, 49.592) (-39.5449, 49.2813) knots 0 0 0 1 2 2 2
  spline S180 degree 2 poles (-39.5449, 49.2813) (-39.9379, 48.9659) (-40.7959, 49.2813) (-41.2983, 49.9074) knots 0 0 0 1 2 2 2
  spline S181 degree 2 poles (-41.2983, 49.9074) (-41.8146, 50.5508) (-41.9205, 51.4445) (-41.5314, 51.7567) knots 0 0 0 1 2 2 2
  spline S182 degree 2 poles (-41.5314, 51.7567) (-41.1403, 52.0706) (-40.2777, 51.7494) (-39.7799, 51.1291) knots 0 0 0 1 2 2 2
  spline S183 degree 2 poles (-39.607, 50.077) (-39.6551, 50.2316) (-39.9072, 50.6247) (-40.1035, 50.8694) knots 0 0 0 1 2 2 2
  spline S184 degree 2 poles (-40.1035, 50.8694) (-40.2999, 51.114) (-40.6275, 51.4433) (-40.773, 51.5261) knots 0 0 0 1 2 2 2
  spline S185 degree 2 poles (-40.773, 51.5261) (-40.9186, 51.6088) (-41.1867, 51.5995) (-41.3196, 51.4928) knots 0 0 0 1 2 2 2
  spline S186 degree 2 poles (-41.3196, 51.4928) (-41.4525, 51.3862) (-41.5235, 51.1233) (-41.4731, 50.9579) knots 0 0 0 1 2 2 2
  spline S187 degree 2 poles (-41.4731, 50.9579) (-41.4239, 50.7979) (-41.1617, 50.4002) (-40.9746, 50.1671) knots 0 0 0 1 2 2 2
  spline S188 degree 2 poles (-40.9746, 50.1671) (-40.7737, 49.9167) (-40.4739, 49.6062) (-40.3187, 49.5154) knots 0 0 0 1 2 2 2
  spline S189 degree 2 poles (-40.3187, 49.5154) (-40.1735, 49.4292) (-39.8954, 49.4339) (-39.7567, 49.5452) knots 0 0 0 1 2 2 2
  spline S190 degree 2 poles (-39.7567, 49.5452) (-39.6257, 49.6503) (-39.5547, 49.9131) (-39.607, 50.077) knots 0 0 0 1 2 2 2
  line L167 (-37.2348, 52.546) -> (-38.1699, 51.8706)
  line L168 (-38.1699, 51.8706) -> (-38.3868, 52.171)
  line L169 (-38.3868, 52.171) -> (-37.4517, 52.8464)
  line L170 (-37.4517, 52.8464) -> (-37.2348, 52.546)
  line L171 (-33.7033, 53.5285) -> (-34.9515, 52.7202)
  line L172 (-34.9515, 52.7202) -> (-35.1206, 52.9815)
  line L173 (-35.1206, 52.9815) -> (-34.6562, 53.2822)
  line L174 (-34.6562, 53.2822) -> (-35.7665, 54.9968)
  line L175 (-35.7665, 54.9968) -> (-36.2309, 54.6961)
  line L176 (-36.2309, 54.6961) -> (-36.3826, 54.9303)
  spline S191 degree 2 poles (-36.3826, 54.9303) (-36.1193, 55.1009) (-35.9672, 55.4112) (-36.0849, 55.6293) knots 0 0 0 1 2 2 2
  line L177 (-36.0849, 55.6293) -> (-35.8195, 55.8012)
  line L178 (-35.8195, 55.8012) -> (-34.3266, 53.4957)
  line L179 (-34.3266, 53.4957) -> (-33.8725, 53.7897)
  line L180 (-33.8725, 53.7897) -> (-33.7033, 53.5285)
  line L181 (-31.6148, 54.7904) -> (-33.2285, 53.8264)
  line L182 (-33.2285, 53.8264) -> (-33.4501, 54.1975)
  spline S192 degree 2 poles (-33.4501, 54.1975) (-33.3738, 54.4646) (-33.2454, 54.9528) (-33.1945, 55.2047) knots 0 0 0 1 2 2 2
  spline S193 degree 2 poles (-33.1945, 55.2047) (-33.0918, 55.712) (-33.109, 56.2369) (-33.2344, 56.4468) knots 0 0 0 1 2 2 2
  spline S194 degree 2 poles (-33.2344, 56.4468) (-33.3003, 56.5571) (-33.467, 56.6819) (-33.5601, 56.6982) knots 0 0 0 1 2 2 2
  spline S195 degree 2 poles (-33.5601, 56.6982) (-33.6533, 56.7145) (-33.8461, 56.6712) (-33.9437, 56.613) knots 0 0 0 1 2 2 2
  spline S196 degree 2 poles (-33.9437, 56.613) (-34.037, 56.5572) (-34.1999, 56.3966) (-34.2653, 56.3086) knots 0 0 0 1 2 2 2
  spline S197 degree 2 poles (-34.2653, 56.3086) (-34.3218, 56.2346) (-34.409, 56.0674) (-34.4337, 56.0124) knots 0 0 0 1 2 2 2
  line L183 (-34.4337, 56.0124) -> (-34.4527, 56.001)
  line L184 (-34.4527, 56.001) -> (-34.6757, 56.3742)
  spline S198 degree 2 poles (-34.6757, 56.3742) (-34.5992, 56.4918) (-34.2732, 56.8275) (-34.0994, 56.9314) knots 0 0 0 1 2 2 2
  spline S199 degree 2 poles (-34.0994, 56.9314) (-33.7325, 57.1505) (-33.0872, 57.0095) (-32.8896, 56.6787) knots 0 0 0 1 2 2 2
  spline S200 degree 2 poles (-32.8896, 56.6787) (-32.7971, 56.5239) (-32.7147, 56.2222) (-32.7124, 56.0739) knots 0 0 0 1 2 2 2
  spline S201 degree 2 poles (-32.7124, 56.0739) (-32.7076, 55.9214) (-32.7578, 55.5864) (-32.795, 55.4175) knots 0 0 0 1 2 2 2
  spline S202 degree 2 poles (-32.795, 55.4175) (-32.8527, 55.1384) (-33.0272, 54.5105) (-33.0809, 54.326) knots 0 0 0 1 2 2 2
  line L185 (-33.0809, 54.326) -> (-31.7959, 55.0936)
  line L186 (-31.7959, 55.0936) -> (-31.6148, 54.7904)
  line L187 (-31.6996, 58.3872) -> (-30.8723, 54.4465)
  line L188 (-30.8723, 54.4465) -> (-31.1745, 54.2783)
  line L189 (-31.1745, 54.2783) -> (-32.0061, 58.2166)
  line L190 (-32.0061, 58.2166) -> (-31.6996, 58.3872)
  line L191 (-28.1875, 56.6299) -> (-29.8574, 55.7669)
  line L192 (-29.8574, 55.7669) -> (-30.0558, 56.1509)
  spline S203 degree 2 poles (-30.0558, 56.1509) (-29.9632, 56.4129) (-29.805, 56.8922) (-29.7387, 57.1406) knots 0 0 0 1 2 2 2
  spline S204 degree 2 poles (-29.7387, 57.1406) (-29.6051, 57.6406) (-29.59, 58.1655) (-29.7023, 58.3828) knots 0 0 0 1 2 2 2
  spline S205 degree 2 poles (-29.7023, 58.3828) (-29.7612, 58.4969) (-29.9199, 58.6317) (-30.0119, 58.6537) knots 0 0 0 1 2 2 2
  spline S206 degree 2 poles (-30.0119, 58.6537) (-30.1039, 58.6757) (-30.299, 58.6444) (-30.3999, 58.5922) knots 0 0 0 1 2 2 2
  spline S207 degree 2 poles (-30.3999, 58.5922) (-30.4965, 58.5423) (-30.669, 58.392) (-30.7397, 58.3082) knots 0 0 0 1 2 2 2
  spline S208 degree 2 poles (-30.7397, 58.3082) (-30.8006, 58.2377) (-30.8979, 58.0763) (-30.9259, 58.0229) knots 0 0 0 1 2 2 2
  line L193 (-30.9259, 58.0229) -> (-30.9457, 58.0127)
  line L194 (-30.9457, 58.0127) -> (-31.1452, 58.3989)
  spline S209 degree 2 poles (-31.1452, 58.3989) (-31.0617, 58.5116) (-30.7157, 58.8266) (-30.5358, 58.9196) knots 0 0 0 1 2 2 2
  spline S210 degree 2 poles (-30.5358, 58.9196) (-30.1561, 59.1158) (-29.5207, 58.9353) (-29.3438, 58.593) knots 0 0 0 1 2 2 2
  spline S211 degree 2 poles (-29.3438, 58.593) (-29.261, 58.4328) (-29.1973, 58.1266) (-29.2042, 57.9785) knots 0 0 0 1 2 2 2
  spline S212 degree 2 poles (-29.2042, 57.9785) (-29.2087, 57.8259) (-29.2794, 57.4947) (-29.3269, 57.3283) knots 0 0 0 1 2 2 2
  spline S213 degree 2 poles (-29.3269, 57.3283) (-29.4017, 57.0534) (-29.6144, 56.4374) (-29.6794, 56.2565) knots 0 0 0 1 2 2 2
  line L195 (-29.6794, 56.2565) -> (-28.3496, 56.9437)
  line L196 (-28.3496, 56.9437) -> (-28.1875, 56.6299)
  line L197 (-26.1219, 57.6119) -> (-27.8219, 56.8098)
  line L198 (-27.8219, 56.8098) -> (-28.0063, 57.2007)
  spline S214 degree 2 poles (-28.0063, 57.2007) (-27.9043, 57.4592) (-27.7289, 57.9325) (-27.6536, 58.1783) knots 0 0 0 1 2 2 2
  spline S215 degree 2 poles (-27.6536, 58.1783) (-27.502, 58.6731) (-27.468, 59.1972) (-27.5723, 59.4183) knots 0 0 0 1 2 2 2
  spline S216 degree 2 poles (-27.5723, 59.4183) (-27.6271, 59.5345) (-27.7808, 59.675) (-27.8719, 59.7003) knots 0 0 0 1 2 2 2
  spline S217 degree 2 poles (-27.8719, 59.7003) (-27.9631, 59.7256) (-28.1592, 59.7013) (-28.2619, 59.6529) knots 0 0 0 1 2 2 2
  spline S218 degree 2 poles (-28.2619, 59.6529) (-28.3602, 59.6065) (-28.5381, 59.4625) (-28.6118, 59.3813) knots 0 0 0 1 2 2 2
  spline S219 degree 2 poles (-28.6118, 59.3813) (-28.6752, 59.3131) (-28.7782, 59.1553) (-28.8082, 59.1029) knots 0 0 0 1 2 2 2
  line L199 (-28.8082, 59.1029) -> (-28.8283, 59.0934)
  line L200 (-28.8283, 59.0934) -> (-29.0138, 59.4866)
  spline S220 degree 2 poles (-29.0138, 59.4866) (-28.9262, 59.5962) (-28.569, 59.8985) (-28.3859, 59.9849) knots 0 0 0 1 2 2 2
  spline S221 degree 2 poles (-28.3859, 59.9849) (-27.9994, 60.1673) (-27.3709, 59.964) (-27.2065, 59.6155) knots 0 0 0 1 2 2 2
  spline S222 degree 2 poles (-27.2065, 59.6155) (-27.1296, 59.4524) (-27.0769, 59.1441) (-27.0891, 58.9963) knots 0 0 0 1 2 2 2
  spline S223 degree 2 poles (-27.0891, 58.9963) (-27.0992, 58.844) (-27.1819, 58.5156) (-27.2354, 58.351) knots 0 0 0 1 2 2 2
  spline S224 degree 2 poles (-27.2354, 58.351) (-27.32, 58.079) (-27.5549, 57.4711) (-27.6263, 57.2926) knots 0 0 0 1 2 2 2
  line L201 (-27.6263, 57.2926) -> (-26.2726, 57.9313)
  line L202 (-26.2726, 57.9313) -> (-26.1219, 57.6119)
  line L203 (-25.8556, 61.1998) -> (-25.4164, 57.1972)
  line L204 (-25.4164, 57.1972) -> (-25.7336, 57.0593)
  line L205 (-25.7336, 57.0593) -> (-26.1773, 61.06)
  line L206 (-26.1773, 61.06) -> (-25.8556, 61.1998)
  line L207 (-22.5315, 59.1085) -> (-24.2776, 58.4124)
  line L208 (-24.2776, 58.4124) -> (-24.4377, 58.8139)
  spline S225 degree 2 poles (-24.4377, 58.8139) (-24.32, 59.0656) (-24.1158, 59.5272) (-24.0256, 59.7679) knots 0 0 0 1 2 2 2
  spline S226 degree 2 poles (-24.0256, 59.7679) (-23.8438, 60.2525) (-23.7776, 60.7735) (-23.8682, 61.0007) knots 0 0 0 1 2 2 2
  spline S227 degree 2 poles (-23.8682, 61.0007) (-23.9158, 61.12) (-24.0605, 61.2697) (-24.1499, 61.3005) knots 0 0 0 1 2 2 2
  spline S228 degree 2 poles (-24.1499, 61.3005) (-24.2393, 61.3313) (-24.4366, 61.3192) (-24.5421, 61.2771) knots 0 0 0 1 2 2 2
  spline S229 degree 2 poles (-24.5421, 61.2771) (-24.6431, 61.2369) (-24.8294, 61.1041) (-24.908, 61.0276) knots 0 0 0 1 2 2 2
  spline S230 degree 2 poles (-24.908, 61.0276) (-24.9755, 60.9634) (-25.088, 60.8122) (-25.1211, 60.7618) knots 0 0 0 1 2 2 2
  line L209 (-25.1211, 60.7618) -> (-25.1418, 60.7536)
  line L210 (-25.1418, 60.7536) -> (-25.3027, 61.1574)
  spline S231 degree 2 poles (-25.3027, 61.1574) (-25.2086, 61.2614) (-24.8335, 61.5412) (-24.6454, 61.6162) knots 0 0 0 1 2 2 2
  spline S232 degree 2 poles (-24.6454, 61.6162) (-24.2484, 61.7744) (-23.6337, 61.5329) (-23.491, 61.175) knots 0 0 0 1 2 2 2
  spline S233 degree 2 poles (-23.491, 61.175) (-23.4242, 61.0075) (-23.3906, 60.6965) (-23.4119, 60.5497) knots 0 0 0 1 2 2 2
  spline S234 degree 2 poles (-23.4119, 60.5497) (-23.4313, 60.3984) (-23.534, 60.0756) (-23.5975, 59.9147) knots 0 0 0 1 2 2 2
  spline S235 degree 2 poles (-23.5975, 59.9147) (-23.6987, 59.6483) (-23.9705, 59.056) (-24.0528, 58.8823) knots 0 0 0 1 2 2 2
  line L211 (-24.0528, 58.8823) -> (-22.6623, 59.4366)
  line L212 (-22.6623, 59.4366) -> (-22.5315, 59.1085)
  spline S236 degree 2 poles (-20.7361, 60.7853) (-20.6621, 60.5783) (-20.6684, 60.1774) (-20.7428, 60.0039) knots 0 0 0 1 2 2 2
  spline S237 degree 2 poles (-20.7428, 60.0039) (-20.8172, 59.8304) (-21.1237, 59.5504) (-21.347, 59.4706) knots 0 0 0 1 2 2 2
  spline S238 degree 2 poles (-21.347, 59.4706) (-21.5517, 59.3975) (-21.9842, 59.3453) (-22.1565, 59.365) knots 0 0 0 1 2 2 2
  line L213 (-22.1565, 59.365) -> (-22.3019, 59.7721)
  line L214 (-22.3019, 59.7721) -> (-22.274, 59.782)
  spline S239 degree 2 poles (-22.274, 59.782) (-22.2182, 59.7653) (-22.0231, 59.7405) (-21.9098, 59.7391) knots 0 0 0 1 2 2 2
  spline S240 degree 2 poles (-21.9098, 59.7391) (-21.7817, 59.7402) (-21.5775, 59.7634) (-21.4589, 59.8058) knots 0 0 0 1 2 2 2
  spline S241 degree 2 poles (-21.4589, 59.8058) (-21.3426, 59.8473) (-21.1538, 60.0092) (-21.1072, 60.1281) knots 0 0 0 1 2 2 2
  spline S242 degree 2 poles (-21.1072, 60.1281) (-21.0658, 60.24) (-21.0728, 60.4945) (-21.1277, 60.648) knots 0 0 0 1 2 2 2
  spline S243 degree 2 poles (-21.1277, 60.648) (-21.1825, 60.8015) (-21.3361, 60.967) (-21.4384, 61.0039) knots 0 0 0 1 2 2 2
  spline S244 degree 2 poles (-21.4384, 61.0039) (-21.5456, 61.0469) (-21.8091, 61.0209) (-21.9557, 60.9686) knots 0 0 0 1 2 2 2
  spline S245 degree 2 poles (-21.9557, 60.9686) (-22.1138, 60.9121) (-22.4104, 60.751) (-22.4983, 60.696) knots 0 0 0 1 2 2 2
  line L215 (-22.4983, 60.696) -> (-23.0269, 62.1753)
  line L216 (-23.0269, 62.1753) -> (-21.4522, 62.738)
  line L217 (-21.4522, 62.738) -> (-21.3317, 62.4007)
  line L218 (-21.3317, 62.4007) -> (-22.5365, 61.9702)
  line L219 (-22.5365, 61.9702) -> (-22.2631, 61.205)
  spline S246 degree 2 poles (-22.2631, 61.205) (-22.1966, 61.2392) (-22.0642, 61.2944) (-22.0084, 61.3143) knots 0 0 0 1 2 2 2
  spline S247 degree 2 poles (-22.0084, 61.3143) (-21.7874, 61.3933) (-21.4569, 61.43) (-21.2792, 61.3729) knots 0 0 0 1 2 2 2
  spline S248 degree 2 poles (-21.2792, 61.3729) (-21.099, 61.3166) (-20.8292, 61.0458) (-20.7361, 60.7853) knots 0 0 0 1 2 2 2
  dimension "Lip_Height" = 2
  dimension "d897" = 116.5
  constraints: 1 centre point, 1 coincident, 1 other
  measures "d897" diameter of A0
extrude "Extrusion31" cut sketch "Sketch48" against normal blind 1 contours L0 L1 L2 L3 L4 L5 L6 L7 | L8 L9 S0 S1 S2 L10 L11 L12 L13 L14 S3 S4 L15 | S5 S6 S7 S8 L16 L17 S9 S10 S11 L18 L19 S12 S13 | L21 S18 S19 L22 L23 L24 L25 L26 S20 S21 L27 | L28 S22 S23 S24 S25 L29 L30 L31 S26 S27 S28 L32 L33 L34 L35 L36 S29 S30 S31 S32 S33 L37 L38 | S34 S35 S36 S37 S38 S39 L39 S40 S41 S42 L40 L41 S43 S44 S45 L42 L43 L44 | L46 L47 L48 L49 | S50 S51 S52 S53 S54 S55 L50 L51 S56 S57 S58 S59 S60 S61 S62 S63 L52 L53 S64 S65 | L54 L55 L56 L57 L58 L59 L60 L61 | L62 L63 L64 L65 | L66 L67 L68 L69 | L70 L71 L72 L73 | L74 L75 S66 S67 S68 L76 L77 L78 L79 L80 S69 S70 L81 | L82 L83 S71 S72 S73 S74 S75 S76 S77 L84 L85 L86 | S82 S83 S84 S85 L88 L89 S86 S87 S88 L90 L91 S89 S90 | L93 S95 S96 L94 L95 L96 L97 L98 S97 S98 L99 | S99 L100 L101 S100 S101 S102 S103 S104 S105 S106 S107 L102 L103 S108 S109 S110 S111 S112 S113 S114 | S115 S116 S117 S118 L104 L105 S119 S120 S121 L106 L107 S122 S123 | S128 S129 S130 S131 L109 S132 S133 S134 S135 S136 L110 L111 L112 S137 S138 L113 L114 | L116 S143 S144 S145 S146 L117 L118 L119 S147 S148 S149 L120 L121 L122 L123 L124 S150 S151 S152 S153 S154 L125 L126 | S155 S156 S157 S158 L127 L128 S159 S160 S161 L129 L130 S162 S163 | L132 L133 S168 S169 S170 L134 L135 L136 L137 L138 S171 S172 L139 | S173 L140 L141 L142 L143 L144 L145 L146 L147 L148 L149 L150 S174 S175 S176 L151 L152 S177 | L153 L154 L155 L156 | L157 L158 L159 L160 L161 L162 S178 L163 L164 L165 L166 | S179 S180 S181 S182 | L167 L168 L169 L170 | L171 L172 L173 L174 L175 L176 S191 L177 L178 L179 L180 | L181 L182 S192 S193 S194 S195 S196 S197 L183 L184 S198 S199 S200 S201 S202 L185 L186 | L187 L188 L189 L190 | L191 L192 S203 S204 S205 S206 S207 S208 L193 L194 S209 S210 S211 S212 S213 L195 L196 | L197 L198 S214 S215 S216 S217 S218 S219 L199 L200 S220 S221 S222 S223 S224 L201 L202 | L203 L204 L205 L206 | L207 L208 S225 S226 S227 S228 S229 S230 L209 L210 S231 S232 S233 S234 S235 L211 L212 | S236 S237 S238 L213 L214 S239 S240 S241 S242 S243 S244 S245 L215 L216 L217 L218 L219 S246 S247 S248
body "Solid1"
